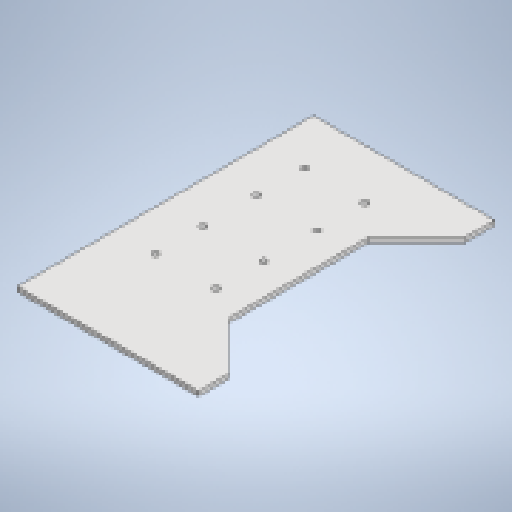
# Autodesk Inventor part: asiura_ita
Saved by Autodesk Inventor 2025.1 (Build 291241000, 241)
## iProperties
Created: 2024-09-04
Part Number: asiura_ita
Material: CFRP
Document SubType Name: Modeling
Designer: right
Density: 1.43 g/cm^3
Appearance: カーボンファイバー
Mass: 10.023 g
Surface Area: 85.0343 cm^2
Volume: 7.00906 cm^3
Author: right
Autodesk Inventor part; units mm, degrees
ref_plane "YZ Plane" through (0, 0, 0) normal (1, 0, 0) x (0, 1, 0)
ref_plane "XZ Plane" through (0, 0, 0) normal (0, 1, 0) x (-1, 0, 0)
ref_plane "XY Plane" through (0, 0, 0) normal (0, 0, 1) x (1, 0, 0)
sketch "スケッチ1" plane through (0, 0, 0) normal (0, 1, 0) x (-1, 0, 0)
  line L0 (30, 49) -> (-30, 49)
  line L1 (-30, 49) -> (-30, -49)
  line L2 (-30, -49) -> (30, -49)
  line L3 (30, -49) -> (30, 49)
  line L4 (30, 49) -> (-30, -49) construction
  line L5 (-30, 49) -> (30, -49) construction
  line L6 (-14, -23) -> (-14, 23)
  line L7 (-14, 23) -> (-30, 39)
  line L8 (-14, -23) -> (-30, -39)
  line L9 (-30, 0) -> (30, 0) construction
  point P0 (0, 0)
  point P1 (-14, 0)
  dimension "d0" = 98
  dimension "d1" = 60
  dimension "d2" = 10
  dimension "d7" = 44
  constraints: 20 end point, 5 midpoint, 2 parallel, 2 perpendicular, 2 point on line, 1 horizontal, 1 horizontal alignment, 1 vertical, 1 other
  measures "d0" distance of L2.end L0.start
  measures "d1" distance of L1.end L2.end
  measures "d2" distance of L1.end L8.end
  measures "d7" distance between parallel lines of L3 L6
extrude "押し出し1" add sketch "スケッチ1" along normal blind 2 contours L3 L2 L1 L8 L6 L7 L0
sketch "スケッチ2" plane through (0, 0, 0) normal (0, -1, 0) x (1, 0, 0)
  arc A0 (-16.0417, 0.3645) -> (-16.0417, 1.6355) centre (-16.5, 1) ccw construction
  arc A1 (3.9583, 0.3645) -> (3.9583, 1.6355) centre (3.5, 1) ccw construction
  arc A2 (-16.0417, -33.1355) -> (-16.0417, -31.8645) centre (-16.5, -32.5) ccw construction
  arc A3 (3.9583, -33.1355) -> (3.9583, -31.8645) centre (3.5, -32.5) ccw construction
  circle A4 centre (-16.5, 1) radius 1.1
  circle A5 centre (3.5, 1) radius 1.1
  circle A6 centre (-16.5, -32.5) radius 1.1
  circle A7 centre (3.5, -32.5) radius 1.1
  line L0 (-16.5, 1) -> (3.5, 1) construction
  line L1 (3.5, 1) -> (3.5, -32.5) construction
  line L2 (3.5, -32.5) -> (-16.5, -32.5) construction
  line L3 (-16.5, -32.5) -> (-16.5, 1) construction
  line L4 (-16.5, 16.75) -> (3.5, 16.75) construction
  line L5 (3.5, 16.75) -> (3.5, -16.75) construction
  line L6 (3.5, -16.75) -> (-16.5, -16.75) construction
  line L7 (-16.5, -16.75) -> (-16.5, 16.75) construction
  line L8 (-30, -49) -> (-30, 49) construction
  circle A8 centre (-16.5, -16.75) radius 1.1
  circle A9 centre (3.5, -16.75) radius 1.1
  circle A10 centre (-16.5, 16.75) radius 1.1
  circle A11 centre (3.5, 16.75) radius 1.1
  point P0 (0, 0)
  point P1 (-16.5, 0)
  point P2 (-30, 0)
  dimension "d8" = 2.2
  dimension "d9" = 2.2
  dimension "d10" = 2.2
  dimension "d11" = 2.2
  dimension "d12" = 2.2
  dimension "d14" = 2.2
  dimension "d15" = 2.2
  constraints: 16 end point, 8 centre point, 8 coincident, 4 parallel, 2 horizontal, 2 midpoint, 2 perpendicular, 2 point on line, 1 collinear, 1 equal radius, 1 horizontal alignment
  measures "d8" diameter of A4
  measures "d9" diameter of A5
  measures "d10" diameter of A6
  measures "d11" diameter of A7
  measures "d12" diameter of A8
  measures "d14" diameter of A10
  measures "d15" diameter of A11
extrude "押し出し2" cut sketch "スケッチ2" against normal through all
fillet "フィレット1" radius 13.25 1 edges at (-30, 1, -49)
sketch "スケッチ3" plane through (0, 0, 0) normal (0, -1, 0) x (1, 0, 0)
  arc A0 (-30, -35.75) -> (-16.75, -49) centre (-16.75, -35.75) ccw projected
  line L0 (30, -49) -> (-16.75, -49) projected
  line L1 (30, -39) -> (30, -49) projected
  line L2 (14, -23) -> (30, -39) projected
  line L3 (14, 23) -> (14, -23) projected
  line L4 (30, 39) -> (14, 23) projected
  line L5 (30, 49) -> (30, 39) projected
  line L6 (-30, 49) -> (30, 49) projected
  line L7 (-30, -35.75) -> (-30, 49) projected
  circle A1 centre (-16.5, 1) radius 1.1 projected
  circle A2 centre (-16.5, -32.5) radius 1.1 projected
  circle A3 centre (3.5, 16.75) radius 1.1 projected
  circle A4 centre (3.5, -16.75) radius 1.1 projected
  circle A5 centre (-16.5, 16.75) radius 1.1 projected
  circle A6 centre (-16.5, -16.75) radius 1.1 projected
  circle A7 centre (3.5, -32.5) radius 1.1 projected
  circle A8 centre (3.5, 1) radius 1.1 projected
  line L8 (-25, 44) -> (25, 44)
  line L9 (25, 44) -> (25, 41.0711)
  line L10 (25, 41.0711) -> (9, 25.0711)
  line L11 (9, 25.0711) -> (9, -25.0711)
  line L12 (9, -25.0711) -> (25, -41.0711)
  line L13 (25, -41.0711) -> (25, -44)
  line L14 (25, -44) -> (-16.75, -44)
  arc A9 (-25, -35.75) -> (-16.75, -44) centre (-16.75, -35.75) ccw
  line L15 (-25, -35.75) -> (-25, 44)
  circle A10 centre (-16.5, -32.5) radius 4
  circle A11 centre (-16.5, -16.75) radius 4
  circle A12 centre (-16.5, 1) radius 4
  circle A13 centre (-16.5, 16.75) radius 4
  circle A14 centre (3.5, 16.75) radius 4
  circle A15 centre (3.5, 1) radius 4
  circle A16 centre (3.5, -16.75) radius 4
  circle A17 centre (3.5, -32.5) radius 4
  line L16 (12, -28.0711) -> (12, -44)
  line L17 (12, 28.0711) -> (12, 44)
  line L18 (-20.5, -32.5) -> (-20.5, 16.75)
  line L19 (-16.5, 20.75) -> (3.5, 20.75)
  line L20 (3.5, 20.75) -> (9, 20.75)
  line L21 (3.5, -36.5) -> (12, -36.5)
  line L22 (3.5, -28.5) -> (12, -28.5)
  line L23 (-16.5, -36.5) -> (3.5, -36.5)
  line L24 (-16.5, -36.5) -> (-24.9658, -36.5)
  line L25 (-16.5, 20.75) -> (-25, 20.75)
  line L26 (-16.5, -28.5) -> (3.5, -28.5)
  line L27 (-0.5, -32.5) -> (-0.5, 16.75)
  line L28 (-12.5, 16.75) -> (-12.5, -32.5)
  line L29 (-16.5, 12.75) -> (3.5, 12.75)
  point P0 (0, 0)
  point P1 (-0.5, 12.75)
  point P2 (-12.5, 12.75)
  point P3 (-12.5, -28.5)
  point P4 (-0.5, -28.5)
  dimension "d19" = 5
  dimension "d20" = 8
  dimension "d21" = 8
  dimension "d22" = 8
  dimension "d23" = 8
  dimension "d24" = 8
  dimension "d25" = 8
  dimension "d26" = 8
  dimension "d27" = 8
  dimension "d28" = 13
  dimension "d29" = 13
  constraints: 44 end point, 18 point on circle, 14 tangent, 10 point on line, 9 centre point, 8 coincident, 5 perpendicular, 2 horizontal, 8 other
  measures "d19" distance between parallel lines of L7 L15
  measures "d20" diameter of A10
  measures "d21" diameter of A11
  measures "d22" diameter of A12
  measures "d23" diameter of A13
  measures "d24" diameter of A14
  measures "d25" diameter of A15
  measures "d26" diameter of A16
  measures "d27" diameter of A17
  measures "d28" distance between parallel lines of L16 L13
  measures "d29" distance from line of L9.end L17
extrude "押し出し3" cut sketch "スケッチ3" against normal through all contours L8 L17 L10 L11 L20 L19 L25 L15 | L24 L23 L21 L16 L14 A9 | L29 L27 L26 L28
sketch "スケッチ4" plane through (0, 0, 0) normal (0, -1, 0) x (1, 0, 0)
  line L0 (-25, 20.75) -> (-25, 44) projected
  line L1 (-25, 44) -> (12, 44) projected
  line L2 (-25, 20.75) -> (12, 44) construction
  line L3 (12, 28.0711) -> (9, 25.0711) projected
  line L4 (9, 25.0711) -> (-25, 44) construction
  line L5 (-25, 21.931) -> (10.1205, 44)
  line L6 (12, 42.819) -> (-23.1205, 20.75)
  line L7 (9, 20.75) -> (-25, 20.75) projected
  line L8 (9.288, 23.7662) -> (-25, 42.8555)
  line L9 (-22.9442, 44) -> (9.7352, 25.8063)
  line L10 (12, 44) -> (12, 28.0711) projected
  line L11 (9, 25.0711) -> (9, 20.75) projected
  point P0 (0, 0)
  point P1 (-7.3439, 33.0257)
  point P2 (-5.3508, 31.9161)
  point P3 (9, 23.9265)
  point P4 (-3.4193, 33.1298)
  point P5 (-5.4124, 34.2395)
  dimension "d32" = 2
  dimension "d33" = 1
  dimension "d34" = 1
  dimension "d35" = 1
  constraints: 12 end point, 7 point on line, 4 parallel
  measures "d32" distance between parallel lines of L6 L5
  measures "d33" distance between parallel lines of L2 L6
  measures "d34" distance between parallel lines of L4 L8
  measures "d35" distance between parallel lines of L9 L4
extrude "押し出し4" add sketch "スケッチ4" against normal up to surface (2 mm away) contours L0 L5 L8 L6 L7 | L0 L1 L9 L5 L8 | L5 L9 L6 L8 | L6 L9 L3 L11 L8 | L5 L1 L10 L6 L9
fillet "フィレット2" radius 3 21 edges at (-24.9658, 1, -36.5) (12, 1, -36.5) (12, 1, -44) (-23.1205, 1, 20.75) (-25, 1, 21.931) (-22.9442, 1, 44) (-25, 1, 42.8555) (-7.3439, 1, 33.0257) (-5.4124, 1, 34.2395) (-3.4193, 1, 33.1298) (-5.3508, 1, 31.9161) (9.7352, 1, 25.8063) (12, 1, 28.0711) (9, 1, 23.9265) (9, 1, 20.75) (12, 1, 42.819) (10.1205, 1, 44) (-12.5, 1, -28.5) (-0.5, 1, -28.5) (-0.5, 1, 12.75) (-12.5, 1, 12.75)
equation "\"d29\" = d28"
equation "\"d33\" = 0.5 * d32"
equation "\"d35\" = d34"
